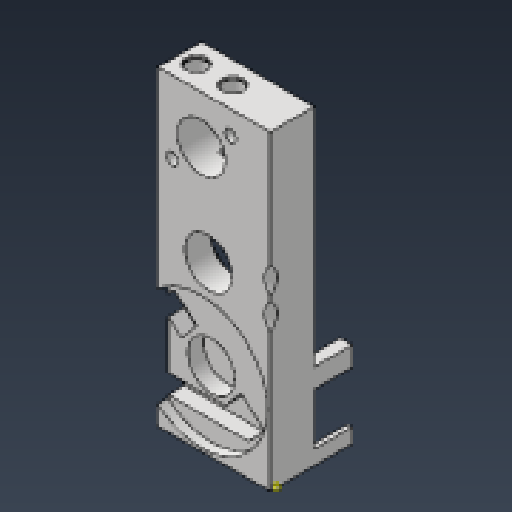
# Autodesk Inventor part: Left_gearbox
Saved by Autodesk Inventor 2026.2 (Build 302298010, 298A)
## iProperties
Created: 2026-04-03
Part Number: Left_gearbox
Material: Generic
Document SubType Name: Modeling
Designer: szymo
Density: 1 g/cm^3
Appearance: Default
Mass: 8.18734 g
Surface Area: 67.5821 cm^2
Volume: 8.18734 cm^3
Author: szymo
Autodesk Inventor part; units mm, degrees
(part 1 of 2)
ref_plane "YZ Plane" through (0, 0, 0) normal (1, 0, 0) x (0, 1, 0)
ref_plane "XZ Plane" through (0, 0, 0) normal (0, 1, 0) x (-1, 0, 0)
ref_plane "XY Plane" through (0, 0, 0) normal (0, 0, 1) x (1, 0, 0)
sketch "Sketch2" plane through (0, 0, 0) normal (0, 0, 1) x (1, 0, 0)
  circle A0 centre (-8.3716, 60.4381) radius 1.0564 construction
  circle A1 centre (-20.6284, 50.1535) radius 1.0564 construction
  circle A2 centre (-14.5, 55.2958) radius 5 projected
  circle A3 centre (-14.5, 55.2958) radius 13.85 construction
  circle A4 centre (-8.9947, 46.9477) radius 1.25 construction
  arc A5 (-9.2865, 53.8165) -> (-9.7521, 54.9117) centre (-14.0905, 52.4209) ccw construction
  arc A6 (-8.9266, 53.8223) -> (-9.2865, 53.8165) centre (-8.9947, 46.9477) ccw construction
  arc A7 (-8.4969, 54.9322) -> (-8.9266, 53.8223) centre (-4.0798, 52.5838) ccw construction
  arc A8 (-8.0797, 54.8952) -> (-8.4969, 54.9322) centre (-8.9947, 46.9477) ccw construction
  arc A9 (-7.852, 53.727) -> (-8.0797, 54.8952) centre (-12.8412, 53.3608) ccw construction
  arc A10 (-7.4988, 53.6579) -> (-7.852, 53.727) centre (-8.9947, 46.9477) ccw construction
  arc A11 (-6.8477, 54.6542) -> (-7.4988, 53.6579) centre (-3.0154, 51.4388) ccw construction
  arc A12 (-6.4474, 54.5312) -> (-6.8477, 54.6542) centre (-8.9947, 46.9477) ccw construction
  arc A13 (-6.4675, 53.3413) -> (-6.4474, 54.5312) centre (-11.4237, 54.0204) ccw construction
  arc A14 (-6.1364, 53.2003) -> (-6.4675, 53.3413) centre (-8.9947, 46.9477) ccw construction
  arc A15 (-5.2924, 54.0394) -> (-6.1364, 53.2003) centre (-2.2123, 50.0975) ccw construction
  arc A16 (-4.9263, 53.8359) -> (-5.2924, 54.0394) centre (-8.9947, 46.9477) ccw construction
  arc A17 (-5.1934, 52.6761) -> (-4.9263, 53.8359) centre (-9.9002, 54.3708) ccw construction
  arc A18 (-4.8988, 52.4693) -> (-5.1934, 52.6761) centre (-8.9947, 46.9477) ccw construction
  arc A19 (-3.8988, 53.1147) -> (-4.8988, 52.4693) centre (-1.7056, 48.6185) ccw construction
  arc A20 (-3.5831, 52.8395) -> (-3.8988, 53.1147) centre (-8.9947, 46.9477) ccw construction
  arc A21 (-4.0855, 51.7606) -> (-3.5831, 52.8395) centre (-8.337, 54.3968) ccw construction
  arc A22 (-3.8403, 51.4971) -> (-4.0855, 51.7606) centre (-8.9947, 46.9477) ccw construction
  arc A23 (-2.728, 51.9204) -> (-3.8403, 51.4971) centre (-1.5175, 47.0665) ccw construction
  arc A24 (-2.4763, 51.5856) -> (-2.728, 51.9204) centre (-8.9947, 46.9477) ccw construction
  arc A25 (-3.1921, 50.6348) -> (-2.4763, 51.5856) centre (-6.8026, 54.0973) ccw construction
  arc A26 (-3.0071, 50.326) -> (-3.1921, 50.6348) centre (-8.9947, 46.9477) ccw construction
  arc A27 (-1.8311, 50.5088) -> (-3.0071, 50.326) centre (-1.6562, 45.5093) ccw construction
  arc A28 (-1.6545, 50.129) -> (-1.8311, 50.5088) centre (-8.9947, 46.9477) ccw construction
  arc A29 (-2.5523, 49.3477) -> (-1.6545, 50.129) centre (-5.364, 53.4853) ccw construction
  arc A30 (-2.4355, 49.0073) -> (-2.5523, 49.3477) centre (-8.9947, 46.9477) ccw construction
  arc A31 (-1.2472, 48.9416) -> (-2.4355, 49.0073) centre (-2.1156, 44.015) ccw construction
  arc A32 (-1.1535, 48.5334) -> (-1.2472, 48.9416) centre (-8.9947, 46.9477) ccw construction
  arc A33 (-2.1941, 47.9558) -> (-1.1535, 48.5334) centre (-4.0841, 52.5876) ccw construction
  arc A34 (-2.1506, 47.5985) -> (-2.1941, 47.9558) centre (-8.9947, 46.9477) ccw construction
  arc A35 (-1.002, 47.2872) -> (-2.1506, 47.5985) centre (-2.8757, 42.6488) ccw construction
  arc A36 (-0.9951, 46.8684) -> (-1.002, 47.2872) centre (-8.9947, 46.9477) ccw construction
  arc A37 (-2.1331, 46.5199) -> (-0.9951, 46.8684) centre (-3.0188, 51.4434) ccw construction
  arc A38 (-2.1649, 46.1613) -> (-2.1331, 46.5199) centre (-8.9947, 46.9477) ccw construction
  arc A39 (-1.106, 45.618) -> (-2.1649, 46.1613) centre (-3.9032, 41.4705) ccw construction
  arc A40 (-1.1864, 45.2069) -> (-1.106, 45.618) centre (-8.9947, 46.9477) ccw construction
  arc A41 (-2.372, 45.1026) -> (-1.1864, 45.2069) centre (-2.2147, 50.1027) ccw construction
  arc A42 (-2.4776, 44.7585) -> (-2.372, 45.1026) centre (-8.9947, 46.9477) ccw construction
  arc A43 (-1.5549, 44.0069) -> (-2.4776, 44.7585) centre (-5.1532, 40.5316) ccw construction
  arc A44 (-1.719, 43.6215) -> (-1.5549, 44.0069) centre (-8.9947, 46.9477) ccw construction
  arc A45 (-2.9003, 43.7659) -> (-1.719, 43.6215) centre (-1.7069, 48.6241) ccw construction
  arc A46 (-3.0752, 43.4513) -> (-2.9003, 43.7659) centre (-8.9947, 46.9477) ccw construction
  arc A47 (-2.3289, 42.5243) -> (-3.0752, 43.4513) centre (-6.5711, 39.8731) ccw construction
  arc A48 (-2.5695, 42.1815) -> (-2.3289, 42.5243) centre (-8.9947, 46.9477) ccw construction
  arc A49 (-3.695, 42.5684) -> (-2.5695, 42.1815) centre (-1.5176, 47.0722) ccw construction
  arc A50 (-3.9314, 42.297) -> (-3.695, 42.5684) centre (-8.9947, 46.9477) ccw construction
  arc A51 (-3.3942, 41.235) -> (-3.9314, 42.297) centre (-8.095, 39.5238) ccw construction
  arc A52 (-3.7009, 40.9498) -> (-3.3942, 41.235) centre (-8.9947, 46.9477) ccw construction
  arc A53 (-4.7213, 41.5622) -> (-3.7009, 40.9498) centre (-1.6551, 45.5149) ccw construction
  arc A54 (-5.009, 41.3459) -> (-4.7213, 41.5622) centre (-8.9947, 46.9477) ccw construction
  arc A55 (-4.7043, 40.1955) -> (-5.009, 41.3459) centre (-9.6581, 39.499) ccw construction
  arc A56 (-5.0636, 39.9802) -> (-4.7043, 40.1955) centre (-8.9947, 46.9477) ccw construction
  arc A57 (-5.9344, 40.7914) -> (-5.0636, 39.9802) centre (-2.1134, 44.0202) ccw construction
  arc A58 (-6.2608, 40.6396) -> (-5.9344, 40.7914) centre (-8.9947, 46.9477) ccw construction
  arc A59 (-6.2019, 39.451) -> (-6.2608, 40.6396) centre (-11.1923, 39.7997) ccw construction
  arc A60 (-6.5981, 39.3151) -> (-6.2019, 39.451) centre (-8.9947, 46.9477) ccw construction
  arc A61 (-7.2812, 40.2896) -> (-6.5981, 39.3151) centre (-2.8724, 42.6535) ccw construction
  arc A62 (-7.632, 40.2091) -> (-7.2812, 40.2896) centre (-8.9947, 46.9477) ccw construction
  arc A63 (-7.8216, 39.0341) -> (-7.632, 40.2091) centre (-12.6304, 40.4128) ccw construction
  arc A64 (-8.2374, 38.9836) -> (-7.8216, 39.0341) centre (-8.9947, 46.9477) ccw construction
  arc A65 (-8.703, 40.0789) -> (-8.2374, 38.9836) centre (-3.899, 41.4744) ccw construction
  arc A66 (-9.0628, 40.073) -> (-8.703, 40.0789) centre (-8.9947, 46.9477) ccw construction
  arc A67 (-9.4925, 38.9632) -> (-9.0628, 40.073) centre (-13.9097, 41.3115) ccw construction
  arc A68 (-9.9097, 39.0002) -> (-9.4925, 38.9632) centre (-8.9947, 46.9477) ccw construction
  arc A69 (-10.1374, 40.1683) -> (-9.9097, 39.0002) centre (-5.1483, 40.5345) ccw construction
  arc A70 (-10.4907, 40.2374) -> (-10.1374, 40.1683) centre (-8.9947, 46.9477) ccw construction
  arc A71 (-11.1417, 39.2411) -> (-10.4907, 40.2374) centre (-14.9741, 42.4565) ccw construction
  arc A72 (-11.5421, 39.3641) -> (-11.1417, 39.2411) centre (-8.9947, 46.9477) ccw construction
  arc A73 (-11.522, 40.554) -> (-11.5421, 39.3641) centre (-6.5657, 39.875) ccw construction
  arc A74 (-11.8531, 40.695) -> (-11.522, 40.554) centre (-8.9947, 46.9477) ccw construction
  arc A75 (-12.6971, 39.8559) -> (-11.8531, 40.695) centre (-15.7772, 43.7978) ccw construction
  arc A76 (-13.0632, 40.0594) -> (-12.6971, 39.8559) centre (-8.9947, 46.9477) ccw construction
  arc A77 (-12.7961, 41.2192) -> (-13.0632, 40.0594) centre (-8.0893, 39.5245) ccw construction
  arc A78 (-13.0907, 41.426) -> (-12.7961, 41.2192) centre (-8.9947, 46.9477) ccw construction
  arc A79 (-14.0906, 40.7807) -> (-13.0907, 41.426) centre (-16.2839, 45.2768) ccw construction
  arc A80 (-14.4064, 41.0558) -> (-14.0906, 40.7807) centre (-8.9947, 46.9477) ccw construction
  arc A81 (-13.904, 42.1347) -> (-14.4064, 41.0558) centre (-9.6525, 39.4985) ccw construction
  arc A82 (-14.1492, 42.3982) -> (-13.904, 42.1347) centre (-8.9947, 46.9477) ccw construction
  arc A83 (-15.2615, 41.9749) -> (-14.1492, 42.3982) centre (-16.472, 46.8288) ccw construction
  arc A84 (-15.5131, 42.3097) -> (-15.2615, 41.9749) centre (-8.9947, 46.9477) ccw construction
  arc A85 (-14.7974, 43.2606) -> (-15.5131, 42.3097) centre (-11.1869, 39.798) ccw construction
  arc A86 (-14.9824, 43.5693) -> (-14.7974, 43.2606) centre (-8.9947, 46.9477) ccw construction
  arc A87 (-16.1584, 43.3865) -> (-14.9824, 43.5693) centre (-16.3333, 48.386) ccw construction
  arc A88 (-16.335, 43.7663) -> (-16.1584, 43.3865) centre (-8.9947, 46.9477) ccw construction
  arc A89 (-15.4372, 44.5476) -> (-16.335, 43.7663) centre (-12.6255, 40.41) ccw construction
  arc A90 (-15.554, 44.888) -> (-15.4372, 44.5476) centre (-8.9947, 46.9477) ccw construction
  arc A91 (-16.7423, 44.9538) -> (-15.554, 44.888) centre (-15.8739, 49.8803) ccw construction
  arc A92 (-16.836, 45.362) -> (-16.7423, 44.9538) centre (-8.9947, 46.9477) ccw construction
  arc A93 (-15.7954, 45.9395) -> (-16.836, 45.362) centre (-13.9054, 41.3077) ccw construction
  arc A94 (-15.8389, 46.2968) -> (-15.7954, 45.9395) centre (-8.9947, 46.9477) ccw construction
  arc A95 (-16.9875, 46.6081) -> (-15.8389, 46.2968) centre (-15.1138, 51.2465) ccw construction
  arc A96 (-16.9944, 47.0269) -> (-16.9875, 46.6081) centre (-8.9947, 46.9477) ccw construction
  arc A97 (-15.8564, 47.3755) -> (-16.9944, 47.0269) centre (-14.9707, 42.452) ccw construction
  arc A98 (-15.8246, 47.734) -> (-15.8564, 47.3755) centre (-8.9947, 46.9477) ccw construction
  arc A99 (-16.8835, 48.2773) -> (-15.8246, 47.734) centre (-14.0863, 52.4248) ccw construction
  arc A100 (-16.8031, 48.6884) -> (-16.8835, 48.2773) centre (-8.9947, 46.9477) ccw construction
  arc A101 (-15.6175, 48.7927) -> (-16.8031, 48.6884) centre (-15.7748, 43.7927) ccw construction
  arc A102 (-15.5119, 49.1368) -> (-15.6175, 48.7927) centre (-8.9947, 46.9477) ccw construction
  arc A103 (-16.4346, 49.8884) -> (-15.5119, 49.1368) centre (-12.8363, 53.3637) ccw construction
  arc A104 (-16.2705, 50.2738) -> (-16.4346, 49.8884) centre (-8.9947, 46.9477) ccw construction
  arc A105 (-15.0892, 50.1294) -> (-16.2705, 50.2738) centre (-16.2826, 45.2713) ccw construction
  arc A106 (-14.9143, 50.444) -> (-15.0892, 50.1294) centre (-8.9947, 46.9477) ccw construction
  arc A107 (-15.6606, 51.371) -> (-14.9143, 50.444) centre (-11.4184, 54.0222) ccw construction
  arc A108 (-15.42, 51.7138) -> (-15.6606, 51.371) centre (-8.9947, 46.9477) ccw construction
  arc A109 (-14.2945, 51.3269) -> (-15.42, 51.7138) centre (-16.4719, 46.8231) ccw construction
  arc A110 (-14.058, 51.5983) -> (-14.2945, 51.3269) centre (-8.9947, 46.9477) ccw construction
  arc A111 (-14.5953, 52.6603) -> (-14.058, 51.5983) centre (-9.8945, 54.3715) ccw construction
  arc A112 (-14.2886, 52.9456) -> (-14.5953, 52.6603) centre (-8.9947, 46.9477) ccw construction
  arc A113 (-13.2682, 52.3331) -> (-14.2886, 52.9456) centre (-16.3344, 48.3804) ccw construction
  arc A114 (-12.9805, 52.5494) -> (-13.2682, 52.3331) centre (-8.9947, 46.9477) ccw construction
  arc A115 (-13.2852, 53.6999) -> (-12.9805, 52.5494) centre (-8.3314, 54.3963) ccw construction
  arc A116 (-12.9259, 53.9151) -> (-13.2852, 53.6999) centre (-8.9947, 46.9477) ccw construction
  arc A117 (-12.0551, 53.1039) -> (-12.9259, 53.9151) centre (-15.8761, 49.8751) ccw construction
  arc A118 (-11.7287, 53.2557) -> (-12.0551, 53.1039) centre (-8.9947, 46.9477) ccw construction
  arc A119 (-11.7876, 54.4443) -> (-11.7287, 53.2557) centre (-6.7972, 54.0957) ccw construction
  arc A120 (-11.3914, 54.5802) -> (-11.7876, 54.4443) centre (-8.9947, 46.9477) ccw construction
  arc A121 (-10.7083, 53.6057) -> (-11.3914, 54.5802) centre (-15.1171, 51.2419) ccw construction
  arc A122 (-10.3575, 53.6863) -> (-10.7083, 53.6057) centre (-8.9947, 46.9477) ccw construction
  arc A123 (-10.1679, 54.8612) -> (-10.3575, 53.6863) centre (-5.3591, 53.4826) ccw construction
  arc A124 (-9.7521, 54.9117) -> (-10.1679, 54.8612) centre (-8.9947, 46.9477) ccw construction
  circle A125 centre (-13, 35.0012) radius 5 projected
  arc A126 (-5.2144, 40.6176) -> (-6.571, 40.1714) centre (-4.0302, 34.7325) ccw construction
  arc A127 (-6.571, 40.1714) -> (-6.8504, 40.5008) centre (-13, 35.0012) ccw construction
  arc A128 (-6.8504, 40.5008) -> (-6.1889, 41.7664) centre (-11.802, 43.8947) ccw construction
  arc A129 (-6.1889, 41.7664) -> (-6.5523, 42.1136) centre (-13, 35.0012) ccw construction
  arc A130 (-6.5523, 42.1136) -> (-7.7864, 41.3951) centre (-4.1704, 36.6033) ccw construction
  arc A131 (-7.7864, 41.3951) -> (-8.1282, 41.6591) centre (-13, 35.0012) ccw construction
  arc A132 (-8.1282, 41.6591) -> (-7.7443, 43.0347) centre (-13.6772, 43.9494) ccw construction
  arc A133 (-7.7443, 43.0347) -> (-8.1719, 43.2988) centre (-13, 35.0012) ccw construction
  arc A134 (-8.1719, 43.2988) -> (-9.2297, 42.3393) centre (-4.6964, 38.4041) ccw construction
  arc A135 (-9.2297, 42.3393) -> (-9.6189, 42.5266) centre (-13, 35.0012) ccw construction
  arc A136 (-9.6189, 42.5266) -> (-9.5294, 43.9519) centre (-15.5228, 43.6131) ccw construction
  arc A137 (-9.5294, 43.9519) -> (-10.0026, 44.1213) centre (-13, 35.0012) ccw construction
  arc A138 (-10.0026, 44.1213) -> (-10.8378, 42.9628) centre (-5.5854, 40.0562) ccw construction
  arc A139 (-10.8378, 42.9628) -> (-11.2574, 43.0651) centre (-13, 35.0012) ccw construction
  arc A140 (-11.2574, 43.0651) -> (-11.4662, 44.4779) centre (-17.2582, 42.9004) ccw construction
  arc A141 (-11.4662, 44.4779) -> (-11.9642, 44.5452) centre (-13, 35.0012) ccw construction
  arc A142 (-11.9642, 44.5452) -> (-12.5404, 43.2384) centre (-6.7984, 41.4873) ccw construction
  arc A143 (-12.5404, 43.2384) -> (-12.9721, 43.2512) centre (-13, 35.0012) ccw construction
  arc A144 (-12.9721, 43.2512) -> (-13.47, 44.5897) centre (-18.8075, 41.8424) ccw construction
  arc A145 (-13.47, 44.5897) -> (-13.9712, 44.5519) centre (-13, 35.0012) ccw construction
  arc A146 (-13.9712, 44.5519) -> (-14.263, 43.1539) centre (-8.2824, 42.6349) ccw construction
  arc A147 (-14.263, 43.1539) -> (-14.688, 43.0767) centre (-13, 35.0012) ccw construction
  arc A148 (-14.688, 43.0767) -> (-15.4533, 44.2824) centre (-20.103, 40.4855) ccw construction
  arc A149 (-15.4533, 44.2824) -> (-15.9357, 44.1413) centre (-13, 35.0012) ccw construction
  arc A150 (-15.9357, 44.1413) -> (-15.9305, 42.7132) centre (-9.9727, 43.4489) ccw construction
  arc A151 (-15.9305, 42.7132) -> (-16.3301, 42.5493) centre (-13, 35.0012) ccw construction
  arc A152 (-16.3301, 42.5493) -> (-17.3293, 43.5696) centre (-21.088, 38.8888) ccw construction
  arc A153 (-17.3293, 43.5696) -> (-17.7718, 43.3312) centre (-13, 35.0012) ccw construction
  arc A154 (-17.7718, 43.3312) -> (-17.4698, 41.9354) centre (-11.7952, 43.8938) ccw construction
  arc A155 (-17.4698, 41.9354) -> (-17.8266, 41.692) centre (-13, 35.0012) ccw construction
  arc A156 (-17.8266, 41.692) -> (-19.0162, 42.4822) centre (-21.7195, 37.1223) ccw construction
  arc A157 (-19.0162, 42.4822) -> (-19.3995, 42.1571) centre (-13, 35.0012) ccw construction
  arc A158 (-19.3995, 42.1571) -> (-18.8139, 40.8545) centre (-13.6704, 43.9499) ccw construction
  arc A159 (-18.8139, 40.8545) -> (-19.1122, 40.5422) centre (-13, 35.0012) ccw construction
  arc A160 (-19.1122, 40.5422) -> (-20.4401, 41.0679) centre (-21.97, 35.263) ccw construction
  arc A161 (-20.4401, 41.0679) -> (-20.7474, 40.6702) centre (-13, 35.0012) ccw construction
  arc A162 (-20.7474, 40.6702) -> (-19.9038, 39.5178) centre (-15.5163, 43.615) ccw construction
  arc A163 (-19.9038, 39.5178) -> (-20.1307, 39.1503) centre (-13, 35.0012) ccw construction
  arc A164 (-20.1307, 39.1503) -> (-21.5389, 39.3884) centre (-21.8284, 33.3924) ccw construction
  arc A165 (-21.5389, 39.3884) -> (-21.7568, 38.9355) centre (-13, 35.0012) ccw construction
  arc A166 (-21.7568, 38.9355) -> (-20.692, 37.9838) centre (-17.2522, 42.9036) ccw construction
  arc A167 (-20.692, 37.9838) -> (-20.8375, 37.5771) centre (-13, 35.0012) ccw construction
  arc A168 (-20.8375, 37.5771) -> (-22.2644, 37.5172) centre (-21.301, 31.592) ccw construction
  arc A169 (-22.2644, 37.5172) -> (-22.3834, 37.0289) centre (-13, 35.0012) ccw construction
  arc A170 (-22.3834, 37.0289) -> (-21.144, 36.3193) centre (-18.8023, 41.8468) ccw construction
  arc A171 (-21.144, 36.3193) -> (-21.2018, 35.8913) centre (-13, 35.0012) ccw construction
  arc A172 (-21.2018, 35.8913) -> (-22.5851, 35.5361) centre (-20.4108, 29.9406) ccw construction
  arc A173 (-22.5851, 35.5361) -> (-22.5999, 35.0337) centre (-13, 35.0012) ccw construction
  arc A174 (-22.5999, 35.0337) -> (-21.2401, 34.5973) centre (-20.0988, 40.4909) ccw construction
  arc A175 (-21.2401, 34.5973) -> (-21.2077, 34.1666) centre (-13, 35.0012) ccw construction
  arc A176 (-21.2077, 34.1666) -> (-22.4868, 33.5315) centre (-19.1967, 28.5104) ccw construction
  arc A177 (-22.4868, 33.5315) -> (-22.3969, 33.037) centre (-13, 35.0012) ccw construction
  arc A178 (-22.3969, 33.037) -> (-20.9761, 32.8929) centre (-21.085, 38.895) ccw construction
  arc A179 (-20.9761, 32.8929) -> (-20.8548, 32.4784) centre (-13, 35.0012) ccw construction
  arc A180 (-20.8548, 32.4784) -> (-21.974, 31.5912) centre (-17.7118, 27.3639) ccw construction
  arc A181 (-21.974, 31.5912) -> (-21.7832, 31.1262) centre (-13, 35.0012) ccw construction
  arc A182 (-21.7832, 31.1262) -> (-20.3634, 31.2807) centre (-21.7179, 37.1289) ccw construction
  arc A183 (-20.3634, 31.2807) -> (-20.1586, 30.9004) centre (-13, 35.0012) ccw construction
  arc A184 (-20.1586, 30.9004) -> (-21.0689, 29.7999) centre (-16.0209, 26.5512) ccw construction
  arc A185 (-21.0689, 29.7999) -> (-20.7856, 29.3848) centre (-13, 35.0012) ccw construction
  arc A186 (-20.7856, 29.3848) -> (-19.429, 29.831) centre (-21.9698, 35.2699) ccw construction
  arc A187 (-19.429, 29.831) -> (-19.1496, 29.5016) centre (-13, 35.0012) ccw construction
  arc A188 (-19.1496, 29.5016) -> (-19.8111, 28.236) centre (-14.198, 26.1077) ccw construction
  arc A189 (-19.8111, 28.236) -> (-19.4477, 27.8888) centre (-13, 35.0012) ccw construction
  arc A190 (-19.4477, 27.8888) -> (-18.2136, 28.6073) centre (-21.8296, 33.3991) ccw construction
  arc A191 (-18.2136, 28.6073) -> (-17.8718, 28.3432) centre (-13, 35.0012) ccw construction
  arc A192 (-17.8718, 28.3432) -> (-18.2557, 26.9677) centre (-12.3228, 26.053) ccw construction
  arc A193 (-18.2557, 26.9677) -> (-17.8281, 26.7036) centre (-13, 35.0012) ccw construction
  arc A194 (-17.8281, 26.7036) -> (-16.7703, 27.6631) centre (-21.3036, 31.5983) ccw construction
  arc A195 (-16.7703, 27.6631) -> (-16.3811, 27.4758) centre (-13, 35.0012) ccw construction
  arc A196 (-16.3811, 27.4758) -> (-16.4706, 26.0505) centre (-10.4772, 26.3893) ccw construction
  arc A197 (-16.4706, 26.0505) -> (-15.9974, 25.8811) centre (-13, 35.0012) ccw construction
  arc A198 (-15.9974, 25.8811) -> (-15.1622, 27.0396) centre (-20.4146, 29.9462) ccw construction
  arc A199 (-15.1622, 27.0396) -> (-14.7426, 26.9373) centre (-13, 35.0012) ccw construction
  arc A200 (-14.7426, 26.9373) -> (-14.5338, 25.5245) centre (-8.7418, 27.102) ccw construction
  arc A201 (-14.5338, 25.5245) -> (-14.0358, 25.4572) centre (-13, 35.0012) ccw construction
  arc A202 (-14.0358, 25.4572) -> (-13.4596, 26.764) centre (-19.2016, 28.5151) ccw construction
  arc A203 (-13.4596, 26.764) -> (-13.0279, 26.7512) centre (-13, 35.0012) ccw construction
  arc A204 (-13.0279, 26.7512) -> (-12.53, 25.4127) centre (-7.1925, 28.16) ccw construction
  arc A205 (-12.53, 25.4127) -> (-12.0288, 25.4504) centre (-13, 35.0012) ccw construction
  arc A206 (-12.0288, 25.4504) -> (-11.737, 26.8485) centre (-17.7176, 27.3675) ccw construction
  arc A207 (-11.737, 26.8485) -> (-11.312, 26.9257) centre (-13, 35.0012) ccw construction
  arc A208 (-11.312, 26.9257) -> (-10.5467, 25.72) centre (-5.897, 29.5169) ccw construction
  arc A209 (-10.5467, 25.72) -> (-10.0643, 25.8611) centre (-13, 35.0012) ccw construction
  arc A210 (-10.0643, 25.8611) -> (-10.0695, 27.2892) centre (-16.0273, 26.5534) ccw construction
  arc A211 (-10.0695, 27.2892) -> (-9.6699, 27.4531) centre (-13, 35.0012) ccw construction
  arc A212 (-9.6699, 27.4531) -> (-8.6707, 26.4328) centre (-4.912, 31.1136) ccw construction
  arc A213 (-8.6707, 26.4328) -> (-8.2282, 26.6712) centre (-13, 35.0012) ccw construction
  arc A214 (-8.2282, 26.6712) -> (-8.5302, 28.067) centre (-14.2048, 26.1086) ccw construction
  arc A215 (-8.5302, 28.067) -> (-8.1734, 28.3104) centre (-13, 35.0012) ccw construction
  arc A216 (-8.1734, 28.3104) -> (-6.9838, 27.5202) centre (-4.2805, 32.8801) ccw construction
  arc A217 (-6.9838, 27.5202) -> (-6.6005, 27.8453) centre (-13, 35.0012) ccw construction
  arc A218 (-6.6005, 27.8453) -> (-7.1861, 29.1479) centre (-12.3296, 26.0525) ccw construction
  arc A219 (-7.1861, 29.1479) -> (-6.8878, 29.4602) centre (-13, 35.0012) ccw construction
  arc A220 (-6.8878, 29.4602) -> (-5.5599, 28.9345) centre (-4.03, 34.7394) ccw construction
  arc A221 (-5.5599, 28.9345) -> (-5.2526, 29.3322) centre (-13, 35.0012) ccw construction
  arc A222 (-5.2526, 29.3322) -> (-6.0962, 30.4845) centre (-10.4837, 26.3874) ccw construction
  arc A223 (-6.0962, 30.4845) -> (-5.8693, 30.8521) centre (-13, 35.0012) ccw construction
  arc A224 (-5.8693, 30.8521) -> (-4.4611, 30.614) centre (-4.1716, 36.61) ccw construction
  arc A225 (-4.4611, 30.614) -> (-4.2432, 31.0669) centre (-13, 35.0012) ccw construction
  arc A226 (-4.2432, 31.0669) -> (-5.308, 32.0186) centre (-8.7478, 27.0988) ccw construction
  arc A227 (-5.308, 32.0186) -> (-5.1625, 32.4253) centre (-13, 35.0012) ccw construction
  arc A228 (-5.1625, 32.4253) -> (-3.7356, 32.4852) centre (-4.699, 38.4104) ccw construction
  arc A229 (-3.7356, 32.4852) -> (-3.6166, 32.9735) centre (-13, 35.0012) ccw construction
  arc A230 (-3.6166, 32.9735) -> (-4.856, 33.6831) centre (-7.1977, 28.1556) ccw construction
  arc A231 (-4.856, 33.6831) -> (-4.7982, 34.1111) centre (-13, 35.0012) ccw construction
  arc A232 (-4.7982, 34.1111) -> (-3.4149, 34.4663) centre (-5.5892, 40.0618) ccw construction
  arc A233 (-3.4149, 34.4663) -> (-3.4001, 34.9687) centre (-13, 35.0012) ccw construction
  arc A234 (-3.4001, 34.9687) -> (-4.7599, 35.4051) centre (-5.9012, 29.5115) ccw construction
  arc A235 (-4.7599, 35.4051) -> (-4.7923, 35.8358) centre (-13, 35.0012) ccw construction
  arc A236 (-4.7923, 35.8358) -> (-3.5132, 36.4709) centre (-6.8033, 41.492) ccw construction
  arc A237 (-3.5132, 36.4709) -> (-3.6031, 36.9654) centre (-13, 35.0012) ccw construction
  arc A238 (-3.6031, 36.9654) -> (-5.0239, 37.1095) centre (-4.915, 31.1074) ccw construction
  arc A239 (-5.0239, 37.1095) -> (-5.1452, 37.524) centre (-13, 35.0012) ccw construction
  arc A240 (-5.1452, 37.524) -> (-4.026, 38.4112) centre (-8.2882, 42.6385) ccw construction
  arc A241 (-4.026, 38.4112) -> (-4.2168, 38.8762) centre (-13, 35.0012) ccw construction
  arc A242 (-4.2168, 38.8762) -> (-5.6366, 38.7217) centre (-4.2821, 32.8735) ccw construction
  arc A243 (-5.6366, 38.7217) -> (-5.8414, 39.102) centre (-13, 35.0012) ccw construction
  arc A244 (-5.8414, 39.102) -> (-4.9311, 40.2025) centre (-9.9791, 43.4512) ccw construction
  arc A245 (-4.9311, 40.2025) -> (-5.2144, 40.6176) centre (-13, 35.0012) ccw construction
  line L0 (0, 0) -> (-23.6, 0)
  line L1 (-23.6, 0) -> (-23.6, 65.2958)
  line L2 (-23.6, 65.2958) -> (0, 65.2958)
  line L3 (0, 65.2958) -> (0, 0)
  circle A246 centre (-13, 35.0012) radius 9.6
  circle A247 centre (-8.9947, 46.9477) radius 8
  line L4 (-14.5, 65.2958) -> (-14.5, 55.2958) construction
  circle A248 centre (-14.5, 55.2958) radius 14.5 construction
  circle A249 centre (-14.5, 14.5) radius 14.5 construction
  line L5 (-14.5, 65.2958) -> (-14.5, 69.7958) construction
  circle A250 centre (-8.9947, 46.9477) radius 8.4
  circle A251 centre (-13, 35.0012) radius 10
  line L6 (-20.7032, 16.4416) -> (-25.4891, 20.4574)
  arc A252 (-22.2751, 24.2876) -> (-25.4891, 20.4574) centre (-14.5, 14.5) ccw
  line L7 (-22.2751, 24.2876) -> (-17.4893, 20.2718)
  arc A253 (-17.4893, 20.2718) -> (-20.7032, 16.4416) centre (-14.5, 14.5) ccw construction
  line L8 (-8.2968, 12.5584) -> (-3.5109, 8.5426)
  arc A254 (-6.7249, 4.7124) -> (-3.5109, 8.5426) centre (-14.5, 14.5) ccw
  line L9 (-6.7249, 4.7124) -> (-11.5107, 8.7282)
  arc A255 (-11.5107, 8.7282) -> (-8.2968, 12.5584) centre (-14.5, 14.5) ccw construction
  line L10 (-17.4893, 20.2718) -> (-20.7032, 16.4416)
  line L11 (-8.2968, 12.5584) -> (-11.5107, 8.7282)
  line L12 (-11.5107, 8.7282) -> (-23.6, 8.7282)
  line L13 (-6.7249, 4.7124) -> (-23.6, 4.7124)
  line L14 (-20.7032, 16.4416) -> (-25.4891, 20.4574)
  arc A256 (-22.2751, 24.2876) -> (-25.4891, 20.4574) centre (-14.5, 14.5) ccw
  line L15 (-22.2751, 24.2876) -> (-17.4893, 20.2718)
  arc A257 (-17.4893, 20.2718) -> (-20.7032, 16.4416) centre (-14.5, 14.5) ccw
  arc A258 (-6.7249, 4.7124) -> (-3.5109, 8.5426) centre (-14.5, 14.5) ccw
  line L16 (-3.5109, 8.5426) -> (-8.2968, 12.5584)
  arc A259 (-11.5107, 8.7282) -> (-8.2968, 12.5584) centre (-14.5, 14.5) ccw
  line L17 (-11.5107, 8.7282) -> (-6.7249, 4.7124)
  line L18 (-19.1651, 20.3726) -> (-22.2701, 22.978) projected
  arc A260 (-22.2701, 22.978) -> (-24.1984, 20.6798) centre (-14.5, 14.5) ccw projected
  line L19 (-24.1984, 20.6798) -> (-21.0934, 18.0744) projected
  arc A261 (-19.1651, 20.3726) -> (-21.0934, 18.0744) centre (-14.5, 14.5) ccw projected
  arc A262 (-6.7299, 6.022) -> (-4.8016, 8.3202) centre (-14.5, 14.5) ccw projected
  line L20 (-4.8016, 8.3202) -> (-7.9066, 10.9256) projected
  arc A263 (-9.8349, 8.6274) -> (-7.9066, 10.9256) centre (-14.5, 14.5) ccw projected
  line L21 (-9.8349, 8.6274) -> (-6.7299, 6.022) projected
  circle A264 centre (-14.5, 14.5) radius 5 projected
  circle A265 centre (-14.5, 14.5) radius 13.85 projected
  circle A266 centre (-8.9947, 46.9477) radius 1.25 construction
  arc A267 (-10.077, 44.3111) -> (-10.0689, 42.8873) centre (-6.4375, 43.62) ccw construction
  arc A268 (-10.4119, 44.475) -> (-10.077, 44.3111) centre (-8.9947, 46.9477) ccw construction
  arc A269 (-11.5409, 43.6075) -> (-10.4119, 44.475) centre (-13.1914, 46.924) ccw construction
  arc A270 (-11.9551, 43.9684) -> (-11.5409, 43.6075) centre (-8.9947, 46.9477) ccw construction
  arc A271 (-11.2503, 45.2055) -> (-11.9551, 43.9684) centre (-8.4439, 42.7872) ccw construction
  arc A272 (-11.4584, 45.5148) -> (-11.2503, 45.2055) centre (-8.9947, 46.9477) ccw construction
  arc A273 (-12.8699, 45.328) -> (-11.4584, 45.5148) centre (-12.641, 49.0255) ccw construction
  arc A274 (-13.0481, 45.8477) -> (-12.8699, 45.328) centre (-8.9947, 46.9477) ccw construction
  arc A275 (-11.8192, 46.5667) -> (-13.0481, 45.8477) centre (-10.5979, 43.0692) ccw construction
  arc A276 (-11.8447, 46.9386) -> (-11.8192, 46.5667) centre (-8.9947, 46.9477) ccw construction
  arc A277 (-13.1605, 47.4826) -> (-11.8447, 46.9386) centre (-11.1136, 50.5703) ccw construction
  arc A278 (-13.0551, 48.0218) -> (-13.1605, 47.4826) centre (-8.9947, 46.9477) ccw construction
  arc A279 (-11.6313, 48.0299) -> (-13.0551, 48.0218) centre (-12.3224, 44.3904) ccw construction
  arc A280 (-11.4674, 48.3648) -> (-11.6313, 48.0299) centre (-8.9947, 46.9477) ccw construction
  arc A281 (-12.335, 49.4938) -> (-11.4674, 48.3648) centre (-9.0184, 51.1443) ccw construction
  arc A282 (-11.974, 49.908) -> (-12.335, 49.4938) centre (-8.9947, 46.9477) ccw construction
  arc A283 (-10.7369, 49.2032) -> (-11.974, 49.908) centre (-13.1552, 46.3968) ccw construction
  arc A284 (-10.4276, 49.4113) -> (-10.7369, 49.2032) centre (-8.9947, 46.9477) ccw construction
  arc A285 (-10.6144, 50.8228) -> (-10.4276, 49.4113) centre (-6.9169, 50.5939) ccw construction
  arc A286 (-10.0947, 51.0011) -> (-10.6144, 50.8228) centre (-8.9947, 46.9477) ccw construction
  arc A287 (-9.3757, 49.7721) -> (-10.0947, 51.0011) centre (-12.8732, 48.5508) ccw construction
  arc A288 (-9.0038, 49.7976) -> (-9.3757, 49.7721) centre (-8.9947, 46.9477) ccw construction
  arc A289 (-8.4598, 51.1135) -> (-9.0038, 49.7976) centre (-5.3721, 49.0665) ccw construction
  arc A290 (-7.9206, 51.008) -> (-8.4598, 51.1135) centre (-8.9947, 46.9477) ccw construction
  arc A291 (-7.9125, 49.5842) -> (-7.9206, 51.008) centre (-11.552, 50.2753) ccw construction
  arc A292 (-7.5776, 49.4204) -> (-7.9125, 49.5842) centre (-8.9947, 46.9477) ccw construction
  arc A293 (-6.4486, 50.2879) -> (-7.5776, 49.4204) centre (-4.7981, 46.9713) ccw construction
  arc A294 (-6.0344, 49.9269) -> (-6.4486, 50.2879) centre (-8.9947, 46.9477) ccw construction
  arc A295 (-6.7392, 48.6898) -> (-6.0344, 49.9269) centre (-9.5456, 51.1081) ccw construction
  arc A296 (-6.5311, 48.3805) -> (-6.7392, 48.6898) centre (-8.9947, 46.9477) ccw construction
  arc A297 (-5.1196, 48.5673) -> (-6.5311, 48.3805) centre (-5.3485, 44.8698) ccw construction
  arc A298 (-4.9413, 48.0476) -> (-5.1196, 48.5673) centre (-8.9947, 46.9477) ccw construction
  arc A299 (-6.1703, 47.3287) -> (-4.9413, 48.0476) centre (-7.3916, 50.8261) ccw construction
  arc A300 (-6.1448, 46.9567) -> (-6.1703, 47.3287) centre (-8.9947, 46.9477) ccw construction
  arc A301 (-4.8289, 46.4127) -> (-6.1448, 46.9567) centre (-6.8759, 43.3251) ccw construction
  arc A302 (-4.9344, 45.8735) -> (-4.8289, 46.4127) centre (-8.9947, 46.9477) ccw construction
  arc A303 (-6.3582, 45.8654) -> (-4.9344, 45.8735) centre (-5.6671, 49.5049) ccw construction
  arc A304 (-6.522, 45.5305) -> (-6.3582, 45.8654) centre (-8.9947, 46.9477) ccw construction
  arc A305 (-5.6545, 44.4015) -> (-6.522, 45.5305) centre (-8.9711, 42.751) ccw construction
  arc A306 (-6.0155, 43.9873) -> (-5.6545, 44.4015) centre (-8.9947, 46.9477) ccw construction
  arc A307 (-7.2526, 44.6921) -> (-6.0155, 43.9873) centre (-4.8343, 47.4985) ccw construction
  arc A308 (-7.5619, 44.484) -> (-7.2526, 44.6921) centre (-8.9947, 46.9477) ccw construction
  arc A309 (-7.3751, 43.0725) -> (-7.5619, 44.484) centre (-11.0726, 43.3014) ccw construction
  arc A310 (-7.8948, 42.8943) -> (-7.3751, 43.0725) centre (-8.9947, 46.9477) ccw construction
  arc A311 (-8.6137, 44.1232) -> (-7.8948, 42.8943) centre (-5.1163, 45.3445) ccw construction
  arc A312 (-8.9857, 44.0977) -> (-8.6137, 44.1232) centre (-8.9947, 46.9477) ccw construction
  arc A313 (-9.5297, 42.7819) -> (-8.9857, 44.0977) centre (-12.6174, 44.8288) ccw construction
  arc A314 (-10.0689, 42.8873) -> (-9.5297, 42.7819) centre (-8.9947, 46.9477) ccw construction
  circle A315 centre (-8.9947, 46.9477) radius 4.2 construction
  circle A316 centre (-8.9947, 46.9477) radius 4.6
  point P0 (-23.6, 5.021)
  point P1 (-23.6, 20.1674)
  point P2 (-16.4204, 43.9712)
  point P3 (-16.1285, 50.5685)
  point P4 (-9.5133, 54.9308)
  point P5 (-4.8639, 40.0967)
  point P6 (-16.9313, 44.196)
  point P7 (-16.5028, 50.7145)
  point P8 (-9.5001, 55.3324)
  point P9 (-4.3207, 39.9681)
  point P10 (-23.6, 23.7912)
  point P11 (-3.7958, 23.2888)
  point P12 (-4.6587, 39.7533)
  point P13 (-9.4902, 38.5623)
  point P14 (-13.6539, 39.9582)
  point P15 (-16.7911, 43.8209)
  point P16 (-23.6, 23.0697)
  point P17 (-23.6, 18.8723)
  point P18 (-16.5599, 44.3461)
  point P19 (-4.5266, 40.3117)
  point P20 (-23.2, 22.4097)
  point P21 (-23.6, 23.0697)
  point P22 (-23.6, 4.0591)
  point P23 (-23.6, 24.9409)
  dimension "d2" = 4.5
  dimension "d14" = 0.4
  dimension "d15" = 0.4
  dimension "d37" = 0.6
  dimension "d121" = 1
  dimension "d122" = 1
  dimension "d123" = 1
  dimension "d124" = 1
  dimension "d125" = 1
  dimension "d126" = 1
  dimension "d127" = 0.4
  constraints: 36 end point, 16 point on circle, 12 centre point, 6 perpendicular, 6 point on line, 3 coincident, 3 concentric, 2 vertical, 1 horizontal, 1 parallel, 1 vertical alignment, 8 other
  measures "d2" distance of L4.start L5.end
  measures "d15" radial gap between concentric circles of A246 A251
  measures "d37" distance edge to line of A251 L1
  measures "d121" distance between parallel lines of L6 L19
  measures "d122" distance between parallel lines of L7 L18
  measures "d123" radial gap between concentric circles of A259 A263
  measures "d124" distance between parallel lines of L8 L20
  measures "d125" distance between parallel lines of L17 L21
  measures "d126" radial gap between concentric circles of A261 A257
ref_plane "Work Plane3" through (-33.4195, -4.4195, -0.6) normal (0, 0, -1) x (-0.5, 0.8660254, 0)
ref_plane "Work Plane4" through (-33.7893, 35.5042, 0.6) normal (0, 0, -1) x (-0.5735764, 0.819152, 0)
ref_plane "Work Plane7" through (-34.0123, 35.7835, 2.1) normal (0, 0, -1) x (-0.6427876, 0.7660444, 0)
extrude "Extrusion3" add sketch "Sketch2" along normal up to surface (2.1 mm away) contours A2 A250 A251 A247 | A2 A250 A251 A265 L1 L2 L3 L0 | A247 A251 A316 A2 | A2 A247 A251 A250 | A251 A247 A246 A250 | A250 A246 A265 A251 | A251 A265 A246 A250 | A250 A246 A247 A251 | A251 A316 A246 A247 | A247 A246 A316 A251 | A250 A125 A246 A265 | A246 A247 A125 A250 | A250 A125 A247 A246 | A246 A316 A247 A125
extrude "Extrusion4" add sketch "Sketch2" against normal blind 1 contours A2 A250 A251 A247 | A2 A250 A251 A265 L1 L2 L3 L0 | A247 A251 A316 A2 | A2 A247 A251 A250 | A251 A247 A246 A250 | A250 A246 A265 A251 | A251 A265 A246 A250 | A250 A246 A247 A251 | A251 A316 A246 A247 | A247 A246 A316 A251 | A250 A125 A246 A265 | A246 A247 A125 A250 | A265 A246 A251 | A251 A265 L1 L13 A254 L8 L11 L12 L6 L10 L7 A252 | A250 A125 A247 A246 | A246 A316 A247 A125 | A265 A246
extrude "Extrusion5" add sketch "Sketch2" against normal blind 3.4 contours A2 A250 A251 A247 | A2 A250 A251 A265 L1 L2 L3 L0 | A247 A251 A316 A2 | A2 A247 A251 A250 | A251 A247 A246 A250 | A250 A246 A265 A251 | A251 A265 A246 A250 | A250 A246 A247 A251 | A251 A316 A246 A247 | A247 A246 A316 A251 | A250 A125 A246 A265 | A246 A247 A125 A250 | A265 A246 A251 | A251 A265 L1 L13 A254 L8 L11 L12 L6 L10 L7 A252 | A250 A125 A247 A246 | A246 A316 A247 A125 | A265 A246
ref_plane "Work Plane5" through (0, 0, -3.4) normal (0, 0, -1) x (-1, 0, 0)